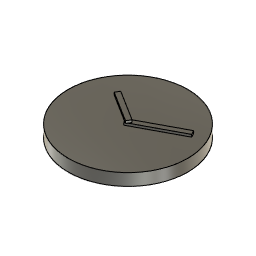
Clock (Autodesk Fusion 360 design; units mm, degrees)
Autodesk Fusion 360 part; units mm, degrees
cylinder "CylinderPrimitive1" add diameter 50 height 5 placed x (1, 0, 0) y (0, 1, 0) z (0, 0, 1) at (0, 0, 0) makes body 1
box "BoxPrimitive1" add length 21 width 2 height 1 placed x (0, 1, 0) y (-1, 0, 0) z (0, 0, 1) at (1, -1, 5) separate body makes body 2
box "BoxPrimitive1'" add length 2 width 15 height 1 placed x (0, -1, 0) y (1, 0, 0) z (0, 0, 1) at (-1, 1, 6) separate body makes body 3 in component "Hour_Hand"
copy_body "Body->Comp1" bodies 2 removing the originals makes body 4 in component "Minutes_Hand"
component "Hour_Hand" placed x (1, 0, 0) y (0, 1, 0) z (0, 0, 1) at (0, 0, 0)
component "Minutes_Hand" placed x (1, 0, 0) y (0, 1, 0) z (0, 0, 1) at (0, 0, 0)
named bodies: "Clock_Face", "Minutes_Hand"
